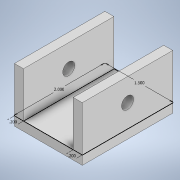
# Autodesk Inventor part: Clip for 1 in 8020
Saved by Autodesk Inventor 2020 (Build 240168000, 168)
## iProperties
Created: 2022-02-15
Part Number: Clip for 1 in 8020
Material: Generic
Document SubType Name: Modeling
Designer: Beaucage
Density: 1 g/cm^3
Appearance: Default
Author: Beaucage
Autodesk Inventor part; units mm, degrees
ref_plane "YZ Plane" through (0, 0, 0) normal (1, 0, 0) x (0, 1, 0)
ref_plane "XZ Plane" through (0, 0, 0) normal (0, 1, 0) x (-1, 0, 0)
ref_plane "XY Plane" through (0, 0, 0) normal (0, 0, 1) x (1, 0, 0)
sketch "Sketch1" plane through (0, 0, 0) normal (0, 1, 0) x (-1, 0, 0)
  line L0 (0, 0) -> (38.1, 0)
  line L1 (38.1, 0) -> (38.1, -50.8)
  line L2 (38.1, -50.8) -> (0, -50.8)
  line L3 (0, -50.8) -> (0, 0)
  line L4 (38.1, -50.8) -> (33.02, -50.8)
  line L5 (33.02, -50.8) -> (33.02, 0)
  line L6 (33.02, 0) -> (38.1, 0)
  line L7 (38.1, 0) -> (38.1, -50.8)
  line L8 (0, -50.8) -> (5.08, -50.8)
  line L9 (5.08, -50.8) -> (5.08, 0)
  line L10 (5.08, 0) -> (0, 0)
  line L11 (0, 0) -> (0, -50.8)
  dimension "d0" = 38.1
  dimension "d1" = 50.8
  dimension "d2" = 5.08
  dimension "d3" = 5.08
  constraints: 24 end point, 6 parallel, 3 horizontal, 3 perpendicular, 2 point on line
  measures "d0" distance of L1.end L2.end
  measures "d1" distance of L0.end L1.end
  measures "d2" distance of L5.end L6.end
  measures "d3" distance of L10.end L9.end
extrude "Extrusion1" add sketch "Sketch1" along normal blind 25.4 contours L0 L9 L2 L3 | L0 L1 L2 L5
extrude "Extrusion2" add sketch "Sketch1" against normal blind 5.08
sketch "Sketch2" plane through (0, 25.4, 0) normal (1, 0, 0) x (0, 0, -1)
  line L0 (50.8, 0) -> (0, 0) projected
  line L1 (25.4, 0) -> (25.4, -12.7)
  point P0 (0, -25.4)
  dimension "d8" = 12.7
  constraints: 2 end point, 1 midpoint, 1 vertical
  measures "d8" distance of L1.start L1.end
hole "Hole1" at (0, 12.7, -25.4) direction (-1, 0, 0) diameter 6.7564 end through all clearance for "Socket Head Cap Screw" size "1/4" standard "Ansi Unified Screw Threads"
body "Solid1"
